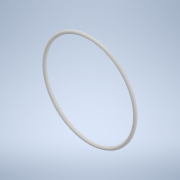
# Autodesk Inventor part: O-Ring_55_2
Saved by Autodesk Inventor 2020.2 (Build 242310000, 310)
## iProperties
Created: 2020-11-13
Part Number: O-Ring_55_2
Material: Generisch
Document SubType Name: Modeling
Designer: g.schardt
Density: 1 g/cm^3
Appearance: Vorgabe
Author: g.schardt
Autodesk Inventor part; units mm, degrees
ref_plane "YZ Plane" through (0, 0, 0) normal (1, 0, 0) x (0, 1, 0)
ref_plane "XZ Plane" through (0, 0, 0) normal (0, 1, 0) x (-1, 0, 0)
ref_plane "XY Plane" through (0, 0, 0) normal (0, 0, 1) x (1, 0, 0)
sketch "Skizze1" plane through (0, 0, 0) normal (1, 0, 0) x (0, 1, 0)
  circle A0 centre (-27.5, 0) radius 1
  line L0 (0, -1.4) -> (0, 1.4) projected
  point P0 (0, 0)
  dimension "d3" = 27.5
  constraints: 1 centre point, 1 horizontal alignment, 1 other
  measures "d3" distance of point (0, 0) A0.centre
revolve "Umdrehung1" add sketch "Skizze1" angle 360 about axis through (0, 0, -10) along (0, 0, 1)
